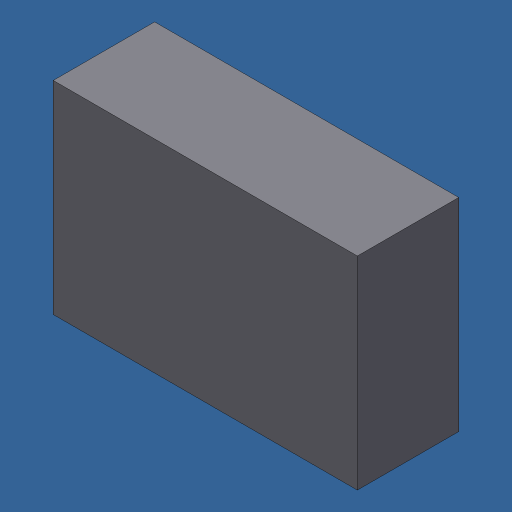
# Autodesk Inventor part: Block, Center Constrained
Saved by Autodesk Inventor 2024.3 (Build 283343000, 343)
## iProperties
Category: _
Manager: _
Created: 2023-11-08
Part Number: Block, Center Constrained
Checked By: 00
Engr Approved By: _
User Status: Work In Process
Material: Steel, MS
Description: BLOCK,CENTER CONSTRAINED
Document SubType Name: Modeling
Mfg Approved By: Stephen.Oerton
Designer: -
Manufacturer: Standard
Standards Organization: Custom
Mass: 772.814 g
Surface Area: 141.935 cm^2
Volume: 98.3224 cm^3
Density: 7.86 g/cm^3
Appearance: Metal-Steel
CN_MASS: 0.77
Width: 2.00 in
Length: 3.00 in
Thickness: 1.00 in
MaterialSize: =<Thickness> X <Width> X <Length>
CN_SERVICEABLE: _
CL_runCount: 0
FIRST_DESCRIPTION: _
SECOND_DESCRIPTION: _
THIRD_DESCRIPTION: _
ModelCat: Uncategorized
ILogicPurgeVersion: 2.2.20.20
OnSaveVersion: 2.2.20.20
Subject: _
Author: -
Keywords: -
Revision Number: A
Autodesk Inventor part; units mm, degrees
ref_plane "YZ Plane" through (0, 0, 0) normal (1, 0, 0) x (0, 1, 0)
ref_plane "XZ Plane" through (0, 0, 0) normal (0, 1, 0) x (-1, 0, 0)
ref_plane "XY Plane" through (0, 0, 0) normal (0, 0, 1) x (1, 0, 0)
sketch "Sketch1" plane through (0, 0, 0) normal (0, 0, 1) x (1, 0, 0)
  line L0 (0, 0) -> (-38.1, 25.4) construction
  line L1 (0, 0) -> (38.1, -25.4) construction
  line L2 (-38.1, 25.4) -> (38.1, 25.4)
  line L3 (38.1, 25.4) -> (38.1, -25.4)
  line L4 (38.1, -25.4) -> (-38.1, -25.4)
  line L5 (-38.1, -25.4) -> (-38.1, 25.4)
  point P0 (0, 0)
  constraints: 12 end point, 3 equal length, 1 coincident, 1 collinear, 1 horizontal, 1 horizontal alignment, 1 perpendicular, 1 vertical alignment
extrude "Extrusion1" add sketch "Sketch1" along normal mid plane 25.4
